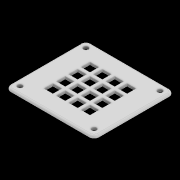
# Autodesk Inventor part: Cubierta Botonera
Saved by Autodesk Inventor 2020 (Build 240168000, 168)
## iProperties
Created: 2022-02-20
Part Number: Cubierta Botonera
Material: Genérico
Document SubType Name: Modeling
Designer: Alférez
Density: 1 g/cm^3
Appearance: Valor por defecto
Author: Alférez
Autodesk Inventor part; units mm, degrees
ref_plane "YZ Plane" through (0, 0, 0) normal (1, 0, 0) x (0, 1, 0)
ref_plane "XZ Plane" through (0, 0, 0) normal (0, 1, 0) x (-1, 0, 0)
ref_plane "XY Plane" through (0, 0, 0) normal (0, 0, 1) x (1, 0, 0)
sketch "Boceto1" plane through (0, 0, 0) normal (0, 1, 0) x (-1, 0, 0)
  line L0 (0, 0) -> (90, 0)
  line L1 (90, 0) -> (90, -80)
  line L2 (90, -80) -> (0, -80)
  line L3 (0, -80) -> (0, 0)
  line L4 (0, 0) -> (17, 0)
  line L5 (17, 0) -> (17, -12)
  line L6 (17, -12) -> (28, -12)
  line L7 (28, -12) -> (28, -23)
  line L8 (28, -23) -> (17, -23)
  line L9 (17, -23) -> (17, -12)
  line L10 (17, -23) -> (17, -27)
  line L11 (17, -27) -> (28, -27)
  line L12 (28, -27) -> (28, -38)
  line L13 (28, -38) -> (17, -38)
  line L14 (17, -38) -> (17, -27)
  line L15 (17, -38) -> (17, -42)
  line L16 (17, -42) -> (28, -42)
  line L17 (28, -42) -> (28, -53)
  line L18 (28, -53) -> (17, -53)
  line L19 (17, -53) -> (17, -42)
  line L20 (17, -53) -> (17, -57)
  line L21 (17, -57) -> (28, -57)
  line L22 (28, -57) -> (28, -68)
  line L23 (28, -68) -> (17, -68)
  line L24 (17, -68) -> (17, -57)
  line L25 (32, -12) -> (43, -12)
  line L26 (43, -12) -> (43, -23)
  line L27 (43, -23) -> (32, -23)
  line L28 (32, -23) -> (32, -12)
  line L29 (32, -23) -> (32, -27)
  line L30 (32, -27) -> (43, -27)
  line L31 (43, -27) -> (43, -38)
  line L32 (43, -38) -> (32, -38)
  line L33 (32, -38) -> (32, -27)
  line L34 (32, -38) -> (32, -42)
  line L35 (32, -42) -> (43, -42)
  line L36 (43, -42) -> (43, -53)
  line L37 (43, -53) -> (32, -53)
  line L38 (32, -53) -> (32, -42)
  line L39 (32, -53) -> (32, -57)
  line L40 (32, -57) -> (43, -57)
  line L41 (43, -57) -> (43, -68)
  line L42 (43, -68) -> (32, -68)
  line L43 (32, -68) -> (32, -57)
  line L44 (43, -12) -> (47, -12)
  line L45 (47, -12) -> (58, -12)
  line L46 (58, -12) -> (58, -23)
  line L47 (58, -23) -> (47, -23)
  line L48 (47, -23) -> (47, -12)
  line L49 (47, -23) -> (47, -27)
  line L50 (47, -27) -> (58, -27)
  line L51 (58, -27) -> (58, -38)
  line L52 (58, -38) -> (47, -38)
  line L53 (47, -38) -> (47, -27)
  line L54 (47, -38) -> (47, -42)
  line L55 (47, -42) -> (58, -42)
  line L56 (58, -42) -> (58, -53)
  line L57 (58, -53) -> (47, -53)
  line L58 (47, -53) -> (47, -42)
  line L59 (47, -53) -> (47, -57)
  line L60 (47, -57) -> (58, -57)
  line L61 (58, -57) -> (58, -68)
  line L62 (58, -68) -> (47, -68)
  line L63 (47, -68) -> (47, -57)
  line L64 (58, -12) -> (62, -12)
  line L65 (73, -23) -> (62, -23)
  line L66 (62, -23) -> (62, -27)
  line L67 (62, -27) -> (73, -27)
  line L68 (73, -12) -> (73, -23)
  line L69 (62, -23) -> (62, -12)
  line L70 (62, -38) -> (62, -27)
  line L71 (62, -38) -> (62, -42)
  line L72 (73, -38) -> (62, -38)
  line L73 (73, -27) -> (73, -38)
  line L74 (62, -12) -> (73, -12)
  line L75 (62, -42) -> (73, -42)
  line L76 (62, -53) -> (62, -42)
  line L77 (73, -42) -> (73, -53)
  line L78 (62, -53) -> (62, -57)
  line L79 (62, -57) -> (73, -57)
  line L80 (62, -68) -> (62, -57)
  line L81 (73, -57) -> (73, -68)
  line L82 (73, -68) -> (62, -68)
  line L83 (73, -53) -> (62, -53)
  line L84 (28, -12) -> (32, -12)
  line L85 (0, 0) -> (8.5, 0)
  line L86 (0, 8.5) -> (0, 0)
  line L87 (0, 0) -> (-8.5, 0)
  line L88 (0, -8.5) -> (0, 0)
  line L89 (0, -80) -> (8.5, -80)
  line L90 (0, -88.5) -> (0, -80)
  line L91 (0, -80) -> (-8.5, -80)
  line L92 (0, -71.5) -> (0, -80)
  line L93 (90, 0) -> (81.5, 0)
  line L94 (90, 8.5) -> (90, 0)
  line L95 (90, 0) -> (98.5, 0)
  line L96 (90, -8.5) -> (90, 0)
  line L97 (90, -80) -> (81.5, -80)
  line L98 (81.5, -80) -> (81.5, -71.5)
  line L99 (90, -80) -> (98.5, -80)
  line L100 (90, -71.5) -> (90, -80)
  circle A0 centre (90, 0) radius 3
  circle A1 centre (90, -80) radius 3
  circle A2 centre (0, 0) radius 3
  circle A3 centre (0, -80) radius 3
  line L101 (0, 0) -> (-8.5, 0)
  line L102 (-8.5, 0) -> (-8.5, 8.5)
  line L103 (-8.5, 8.5) -> (0, 8.5)
  line L104 (0, 8.5) -> (0, 0)
  line L105 (0, -88.5) -> (-8.5, -88.5)
  line L106 (-8.5, -88.5) -> (-8.5, -80)
  line L107 (-8.5, -80) -> (0, -80)
  line L108 (0, -80) -> (0, -88.5)
  line L109 (98.5, 0) -> (90, 0)
  line L110 (90, 0) -> (90, 8.5)
  line L111 (90, 8.5) -> (98.5, 8.5)
  line L112 (98.5, 8.5) -> (98.5, 0)
  line L113 (98.5, -88.5) -> (90, -88.5)
  line L114 (90, -88.5) -> (90, -80)
  line L115 (90, -80) -> (98.5, -80)
  line L116 (98.5, -80) -> (98.5, -88.5)
  line L117 (98.5, 8.5) -> (-8.5, 8.5)
  line L118 (-8.5, 8.5) -> (-8.5, -88.5)
  line L119 (-8.5, -88.5) -> (98.5, -88.5)
  line L120 (98.5, -88.5) -> (98.5, 8.5)
  dimension "d0" = 90
  dimension "d1" = 80
  dimension "d2" = 17
  dimension "d3" = 12
  dimension "d4" = 11
  dimension "d5" = 11
  dimension "d6" = 4
  dimension "d7" = 11
  dimension "d8" = 11
  dimension "d9" = 4
  dimension "d10" = 11
  dimension "d11" = 11
  dimension "d12" = 4
  dimension "d13" = 11
  dimension "d14" = 11
  dimension "d16" = 11
  dimension "d17" = 11
  dimension "d18" = 4
  dimension "d19" = 11
  dimension "d20" = 11
  dimension "d21" = 4
  dimension "d22" = 11
  dimension "d23" = 11
  dimension "d24" = 4
  dimension "d25" = 11
  dimension "d26" = 11
  dimension "d27" = 4
  dimension "d28" = 11
  dimension "d29" = 11
  dimension "d30" = 4
  dimension "d31" = 11
  dimension "d32" = 11
  dimension "d33" = 4
  dimension "d34" = 11
  dimension "d35" = 11
  dimension "d36" = 4
  dimension "d37" = 11
  dimension "d38" = 11
  dimension "d39" = 4
  dimension "d40" = 11
  dimension "d41" = 11
  dimension "d42" = 4
  dimension "d43" = 11
  dimension "d44" = 11
  dimension "d45" = 4
  dimension "d46" = 11
  dimension "d47" = 11
  dimension "d48" = 4
  dimension "d49" = 11
  dimension "d50" = 11
  dimension "d51" = 4
  dimension "d52" = 8.5
  dimension "d53" = 8.5
  dimension "d54" = 8.5
  dimension "d55" = 8.5
  dimension "d56" = 8.5
  dimension "d57" = 8.5
  dimension "d58" = 8.5
  dimension "d59" = 6
  dimension "d60" = 6
  dimension "d61" = 6
  dimension "d62" = 8.5
  dimension "d63" = 8.5
  dimension "d64" = 8.5
  constraints: 242 end point, 52 equal length, 29 horizontal, 27 perpendicular, 12 vertical, 4 centre point, 4 coincident, 1 point on line
  measures "d0" distance of L1.end L2.end
  measures "d1" distance of L0.end L1.end
  measures "d2" distance of L0.start L4.end
  measures "d3" distance of L4.end L5.end
  measures "d4" distance of L7.end L8.end
  measures "d5" distance of L6.end L7.end
  measures "d6" distance of L8.end L10.end
  measures "d7" distance of L12.end L13.end
  measures "d8" distance of L11.end L12.end
  measures "d9" distance of L13.end L15.end
  measures "d10" distance of L17.end L18.end
  measures "d11" distance of L16.end L17.end
  measures "d12" distance of L18.end L20.end
  measures "d13" distance of L22.end L23.end
  measures "d14" distance of L21.end L22.end
  measures "d16" distance of L27.start L27.end
  measures "d17" distance of L26.start L27.start
  measures "d18" distance of L27.end L29.end
  measures "d19" distance of L32.start L33.start
  measures "d20" distance of L30.end L32.start
  measures "d21" distance of L33.start L34.end
  measures "d22" distance of L36.end L38.start
  measures "d23" distance of L35.end L36.end
  measures "d24" distance of L38.start L39.end
  measures "d25" distance of L41.end L43.start
  measures "d26" distance of L40.end L41.end
  measures "d27" distance of L26.start L44.end
  measures "d28" distance of L47.start L49.start
  measures "d29" distance of L46.start L47.start
  measures "d30" distance of L49.start L53.end
  measures "d31" distance of L52.start L53.start
  measures "d32" distance of L50.end L52.start
  measures "d33" distance of L53.start L54.end
  measures "d34" distance of L57.start L58.start
  measures "d35" distance of L55.end L57.start
  measures "d36" distance of L58.start L59.end
  measures "d37" distance of L61.end L62.end
  measures "d38" distance of L60.end L61.end
  measures "d39" distance of L46.start L64.end
  measures "d40" distance of L68.end L66.start
  measures "d41" distance of L68.start L68.end
  measures "d42" distance of L66.start L66.end
  measures "d43" distance of L72.start L70.start
  measures "d44" distance of L67.end L72.start
  measures "d45" distance of L70.start L76.end
  measures "d46" distance of L83.start L78.start
  measures "d47" distance of L77.start L83.start
  measures "d48" distance of L78.start L80.end
  measures "d49" distance of L81.end L82.end
  measures "d50" distance of L81.start L81.end
  measures "d51" distance of L6.end L84.end
  measures "d52" distance of L86.end L87.end
  measures "d53" distance of L86.start L86.end
  measures "d54" distance of L91.end L90.end
  measures "d55" distance of L90.end L90.start
  measures "d56" distance of L95.end L94.end
  measures "d57" distance of L94.end L94.start
  measures "d58" distance of L99.start L99.end
  measures "d59" diameter of A0
  measures "d60" diameter of A1
  measures "d61" diameter of A2
  measures "d62" distance of L102.end L103.end
  measures "d63" distance of L101.end L102.end
  measures "d64" distance of L106.end L108.start
extrude "Extrusión1" add sketch "Boceto1" along normal blind 3 contours A2 L86 L117 L94 A0 L0 | L0 A0 L1 A1 L2 A3 L3 A2 | L3 A3 L91 L118 L87 A2 | A2 L87 L102 L103 L86 | L111 L112 L95 A0 L94 | L91 A3 L90 L105 L106 | L2 A1 L114 L119 L90 A3 | L95 L120 L99 A1 L1 A0 | L116 L113 L114 A1 L99
fillet "Empalme1" radius 6 4 edges at (-98.5, 1.5, 8.5) (-98.5, 1.5, -88.5) (8.5, 1.5, 8.5) (8.5, 1.5, -88.5)
fillet "Empalme2" radius 2 8 edges at (-96.7426, 3, -86.7426) (-98.5, 3, 1.25) (-96.7426, 3, 6.7426) (1.25, 3, 8.5) (6.7426, 3, 6.7426) (8.5, 3, 1.25) (6.7426, 3, -86.7426) (1.25, 3, -88.5)
